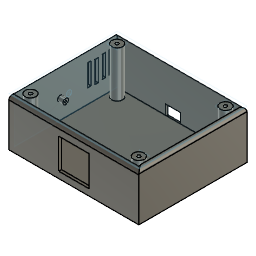
Electronics_Enclosure_Tub (Autodesk Fusion 360 design; units mm, degrees)
Autodesk Fusion 360 part; units mm, degrees
note: some values were not read from the file. Chosen so that the rebuilt part matches the saved one: which pieces of a blend or face edit are solid.
sketch "Sketch1" plane through (0, 0, 0) normal (0, 0, 1) x (1, 0, 0)
  line L0 (0, 0) -> (120, 0)
  line L1 (120, 0) -> (120, 100)
  line L2 (120, 100) -> (0, 100)
  line L3 (0, 100) -> (0, 0)
  dimension "d1" = 120
  dimension "d2" = 100
  constraint horizontal L0
  constraint vertical L1
  constraint horizontal L2
  constraint vertical L3
  constraint coincident L0.start L3.end
  measures "d1" distance of L1.end L2.end
  measures "d2" distance of L0.start L2.end
extrude "Extrude1" add sketch "Sketch1" along normal blind 45
sketch "Sketch2" plane through (0, 0, 45) normal (0, 0, 1) x (-1, 0, 0)
  line L0 (0, -100) -> (0, 0)
  line L1 (0, 0) -> (-120, 0)
  line L2 (-120, 0) -> (-120, -100)
  line L3 (-120, -100) -> (0, -100)
shell "Shell1" thickness 2.5 removed faces 1 at (40, 33.3333, 45)
fillet "Fillet1" radius 5 4 edges at (60, 0, 45) (120, 50, 45) (0, 50, 45) (60, 100, 45)
sketch "Sketch3" plane through (0, 0, 45) normal (0, 0, 1) x (-1, 0, 0)
  circle A0 centre (-110, -10) radius 5
  circle A1 centre (-10, -10) radius 5
  circle A2 centre (-110, -90) radius 5
  circle A3 centre (-10, -90) radius 5
  dimension "d8" = 10
  dimension "d9" = 10
  measures "d8" diameter of A0
  measures "d9" diameter of A3
extrude "Extrude2" add sketch "Sketch3" against normal blind 42.5
hole "Hole1" at (10, 90, 45) direction (0, 0, -1) diameter 3 depth 15 tip angle 90
hole "Hole2" at (10, 10, 45) direction (0, 0, -1) diameter 3 depth 15 tip angle 90
hole "Hole3" at (110.1155, 10.028, 45) direction (0, 0, -1) diameter 3 depth 15 tip angle 90
hole "Hole4" at (110, 90, 45) direction (0, 0, -1) diameter 3 depth 15 tip angle 90
sketch "Sketch4" plane through (0, 0, 0) normal (0, -1, 0) x (1, 0, 0)
  line L0 (120, 40) -> (0, 40)
  line L1 (0, 40) -> (0, 0)
  line L2 (0, 0) -> (120, 0)
  line L3 (120, 0) -> (120, 40)
  line L4 (46, 34) -> (74, 34)
  line L5 (74, 34) -> (74, 6)
  line L6 (74, 6) -> (46, 6)
  line L7 (46, 6) -> (46, 34)
  dimension "d24" = 28
  dimension "d25" = 28
  dimension "d26" = 46
  dimension "d27" = 6
  constraint horizontal L4
  constraint vertical L5
  constraint horizontal L6
  constraint vertical L7
  measures "d24" distance of L4.start L6.end
  measures "d25" distance of L4.start L4.end
  measures "d26" distance of L1 L7
  measures "d27" distance of L0 L4
extrude "Extrude3" cut sketch "Sketch4" against normal blind 2.5 contours L4 L5 L6 L7
sketch "Sketch5" plane through (0, 100, 0) normal (0, 1, 0) x (-1, 0, 0)
  line L0 (0, 40) -> (-120, 40)
  line L1 (-120, 40) -> (-120, 0)
  line L2 (-120, 0) -> (0, 0)
  line L3 (0, 0) -> (0, 40)
  line L4 (-60.8692, 1.5) -> (-46.8692, 1.5)
  line L5 (-46.8692, 1.5) -> (-46.8692, 11.5)
  line L6 (-46.8692, 11.5) -> (-60.8692, 11.5)
  line L7 (-60.8692, 11.5) -> (-60.8692, 1.5)
  dimension "d30" = 10
  dimension "d31" = 14
  dimension "d32" = 1.5
  constraint horizontal L4
  constraint vertical L5
  constraint horizontal L6
  constraint vertical L7
  measures "d30" distance of L4.end L5.end
  measures "d31" distance of L5.end L6.end
  measures "d32" distance of L2 L4
extrude "Extrude4" cut sketch "Sketch5" against normal blind 2.5 contours L4 L5 L6 L7
sketch "Sketch6" plane through (0, 0, 0) normal (-1, 0, 0) x (0, -1, 0)
  line L0 (-0.0451, 40.6699) -> (-99.9549, 40.6699)
  arc A0 (-99.9549, 40.6699) -> (-100, 40) centre (-95, 40) ccw
  line L1 (-100, 40) -> (-100, 0)
  line L2 (-100, 0) -> (0, 0)
  line L3 (0, 0) -> (0, 40)
  arc A1 (0, 40) -> (-0.0451, 40.6699) centre (-5, 40) ccw
  line L4 (-93.0228, 36.1358) -> (-90.0228, 36.1358)
  line L5 (-90.0228, 36.1358) -> (-90.0228, 16.1358)
  line L6 (-90.0228, 16.1358) -> (-93.0228, 16.1358)
  line L7 (-93.0228, 16.1358) -> (-93.0228, 36.1358)
  dimension "d35" = 20
  dimension "d36" = 3
  constraint horizontal L4
  constraint vertical L5
  constraint horizontal L6
  constraint vertical L7
  measures "d35" distance of L4.end L5.end
  measures "d36" distance of L4.start L4.end
extrude "Extrude5" cut sketch "Sketch6" against normal blind 2.5 contours L4 L5 L6 L7
sketch "Sketch7" plane through (0, 0, 0) normal (-1, 0, 0) x (0, -1, 0)
  line L0 (-90.0228, 36.1358) -> (-90.0228, 16.1358)
  line L1 (-90.0228, 16.1358) -> (-93.0228, 16.1358)
  line L2 (-93.0228, 16.1358) -> (-93.0228, 36.1358)
  line L3 (-93.0228, 36.1358) -> (-90.0228, 36.1358)
  line L4 (-0.0451, 40.6699) -> (-99.9549, 40.6699)
  arc A0 (-99.9549, 40.6699) -> (-100, 40) centre (-95, 40) ccw
  line L5 (-100, 40) -> (-100, 0)
  line L6 (-100, 0) -> (0, 0)
  line L7 (0, 0) -> (0, 40)
  arc A1 (0, 40) -> (-0.0451, 40.6699) centre (-5, 40) ccw
  line L8 (-86.9191, 35.754) -> (-83.9191, 35.754)
  line L9 (-83.9191, 35.754) -> (-83.9191, 15.754)
  line L10 (-83.9191, 15.754) -> (-86.9191, 15.754)
  line L11 (-86.9191, 15.754) -> (-86.9191, 35.754)
  line L12 (-80, 35) -> (-77, 35)
  line L13 (-77, 35) -> (-77, 15)
  line L14 (-77, 15) -> (-80, 15)
  line L15 (-80, 15) -> (-80, 35)
  line L16 (-73.3573, 35.754) -> (-70.3573, 35.754)
  line L17 (-70.3573, 35.754) -> (-70.3573, 15.754)
  line L18 (-70.3573, 15.754) -> (-73.3573, 15.754)
  line L19 (-73.3573, 15.754) -> (-73.3573, 35.754)
  dimension "d39" = 20
  dimension "d40" = 3
  dimension "d41" = 3
  dimension "d42" = 20
  dimension "d43" = 20
  dimension "d44" = 3
  constraint horizontal L8
  constraint vertical L9
  constraint horizontal L10
  constraint vertical L11
  constraint horizontal L12
  constraint vertical L13
  constraint horizontal L14
  constraint vertical L15
  constraint horizontal L16
  constraint vertical L17
  constraint horizontal L18
  constraint vertical L19
  measures "d39" distance of L8.end L9.end
  measures "d40" distance of L8.start L8.end
  measures "d41" distance of L12.start L12.end
  measures "d42" distance of L12.end L13.end
  measures "d43" distance of L16.end L17.end
  measures "d44" distance of L16.start L16.end
extrude "Extrude6" cut sketch "Sketch7" against normal blind 2.5 contours L8 L9 L10 L11 | L12 L13 L14 L15 | L16 L17 L18 L19
sketch "Sketch8" plane through (2.5, 0, 0) normal (1, 0, 0) x (0, 1, 0)
  line L0 (83.9191, 15.754) -> (83.9191, 35.754)
  line L1 (83.9191, 35.754) -> (86.9191, 35.754)
  line L2 (86.9191, 35.754) -> (86.9191, 15.754)
  line L3 (86.9191, 15.754) -> (83.9191, 15.754)
  line L4 (77, 15) -> (77, 35)
  line L5 (77, 35) -> (80, 35)
  line L6 (80, 35) -> (80, 15)
  line L7 (80, 15) -> (77, 15)
  line L8 (70.3573, 15.754) -> (70.3573, 35.754)
  line L9 (70.3573, 35.754) -> (73.3573, 35.754)
  line L10 (73.3573, 35.754) -> (73.3573, 15.754)
  line L11 (73.3573, 15.754) -> (70.3573, 15.754)
  line L12 (90.0228, 16.1358) -> (90.0228, 36.1358)
  line L13 (90.0228, 36.1358) -> (93.0228, 36.1358)
  line L14 (93.0228, 36.1358) -> (93.0228, 16.1358)
  line L15 (93.0228, 16.1358) -> (90.0228, 16.1358)
  arc A0 (97.5, 44.3301) -> (95, 45) centre (95, 40) ccw
  line L16 (95, 45) -> (5, 45)
  arc A1 (5, 45) -> (2.5, 44.3301) centre (5, 40) ccw
  line L17 (2.5, 44.3301) -> (2.5, 2.5)
  line L18 (2.5, 2.5) -> (97.5, 2.5)
  line L19 (97.5, 2.5) -> (97.5, 44.3301)
sketch "Sketch9" plane through (0, 0, 0) normal (-1, 0, 0) x (0, -1, 0)
  line L0 (-83.9191, 35.754) -> (-83.9191, 15.754)
  line L1 (-83.9191, 15.754) -> (-86.9191, 15.754)
  line L2 (-86.9191, 15.754) -> (-86.9191, 35.754)
  line L3 (-86.9191, 35.754) -> (-83.9191, 35.754)
  line L4 (-77, 35) -> (-77, 15)
  line L5 (-77, 15) -> (-80, 15)
  line L6 (-80, 15) -> (-80, 35)
  line L7 (-80, 35) -> (-77, 35)
  line L8 (-70.3573, 35.754) -> (-70.3573, 15.754)
  line L9 (-70.3573, 15.754) -> (-73.3573, 15.754)
  line L10 (-73.3573, 15.754) -> (-73.3573, 35.754)
  line L11 (-73.3573, 35.754) -> (-70.3573, 35.754)
  line L12 (-90.0228, 36.1358) -> (-90.0228, 16.1358)
  line L13 (-90.0228, 16.1358) -> (-93.0228, 16.1358)
  line L14 (-93.0228, 16.1358) -> (-93.0228, 36.1358)
  line L15 (-93.0228, 36.1358) -> (-90.0228, 36.1358)
  line L16 (-0.0451, 40.6699) -> (-99.9549, 40.6699)
  arc A0 (-99.9549, 40.6699) -> (-100, 40) centre (-95, 40) ccw
  line L17 (-100, 40) -> (-100, 0)
  line L18 (-100, 0) -> (0, 0)
  line L19 (0, 0) -> (0, 40)
  arc A1 (0, 40) -> (-0.0451, 40.6699) centre (-5, 40) ccw
  circle A2 centre (-45, 20) radius 2.5
  circle A3 centre (-45, 20) radius 1
  dimension "d47" = 5
  dimension "d48" = 2
  constraint concentric A2 A3
  measures "d47" diameter of A2
  measures "d48" diameter of A3
extrude "Extrude7" add sketch "Sketch9" against normal blind 7.5 contours A2
